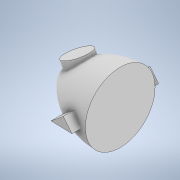
# Autodesk Inventor part: 1
Saved by Autodesk Inventor 2021.1 (Build 251245010, 245A)
## iProperties
Created: 2023-10-12
Part Number: 1
Material: Типовые
Document SubType Name: Modeling
Designer: Lenovo
Density: 1 g/cm^3
Appearance: По умолчанию
Author: Lenovo
Autodesk Inventor part; units mm, degrees
ref_plane "YZ Plane" through (0, 0, 0) normal (1, 0, 0) x (0, 1, 0)
ref_plane "XZ Plane" through (0, 0, 0) normal (0, 1, 0) x (-1, 0, 0)
ref_plane "XY Plane" through (0, 0, 0) normal (0, 0, 1) x (1, 0, 0)
sketch "Эскиз1" plane through (0, 0, 0) normal (0, 1, 0) x (-1, 0, 0)
  line L0 (0, 0) -> (0, -60)
  arc A0 (0, -60) -> (103.923, 0) centre (0, 60) ccw
  line L1 (103.923, 0) -> (0, 0)
  dimension "d0" = 60
  constraints: 4 end point, 2 point on circle, 1 centre point, 1 perpendicular, 1 vertical
  measures "d0" distance of L0.start L0.end
revolve "Вращение1" add sketch "Эскиз1" angle 360 about axis through (-103.923, 0, 0) along (1, 0, 0)
sketch "Эскиз2" plane through (0, 0, 0) normal (0, 0, 1) x (1, 0, 0)
  line L0 (-23.2081, 12.324) -> (-44.4377, -4.9629)
  line L1 (-44.4377, -4.9629) -> (-8.2356, -6.0633)
  line L2 (-8.2356, -6.0633) -> (-23.2081, 12.324)
  point P0 (0, 0)
  constraints: 6 end point, 1 perpendicular
extrude "Выдавливание1" add sketch "Эскиз2" along normal mid plane 149.25 separate body
sketch "Эскиз3" plane through (0, 0, 0) normal (0, 0, 1) x (1, 0, 0)
  line L0 (-52.5078, 0) -> (-32.1747, 10.0687)
  line L1 (-32.1747, 10.0687) -> (-53.7333, 53.6048)
  line L2 (-53.7333, 53.6048) -> (-74.0664, 43.5361)
  line L3 (-52.5078, 0) -> (-74.0664, 43.5361)
  point P0 (0, 0)
  constraints: 8 end point, 3 perpendicular
revolve "Вращение2" add sketch "Эскиз3" angle 360 about axis through (-52.5078, 0, 0) along (-0.4437612, 0.8961451, 0) separate body
sketch "Эскиз4" plane through (0, 0, 0) normal (0, 0, 1) x (1, 0, 0)
  arc A0 (-88.153, -26.4746) -> (-22.9883, -26.4746) centre (-55.5707, -26.4746) ccw
  line L0 (-22.9883, -26.4746) -> (-88.153, -26.4746)
  point P0 (0, 0)
  constraints: 2 end point, 2 point on circle, 1 centre point
revolve "Вращение3" add sketch "Эскиз4" angle 360 about axis through (-22.9883, -26.4746, 0) along (-1, 0, 0) separate body
